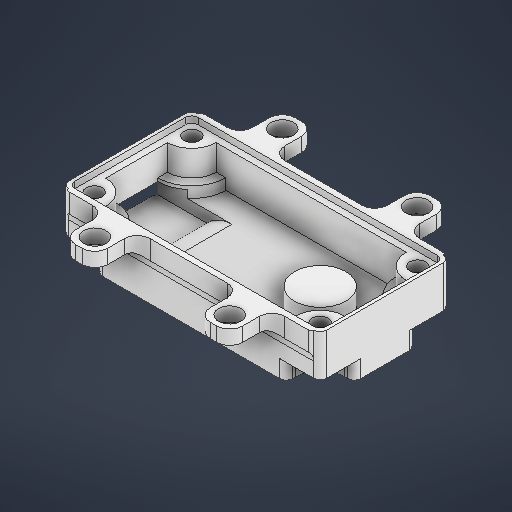
# Autodesk Inventor part: ServoCase
Saved by Autodesk Inventor 2026.2 (Build 302298010, 298A)
## iProperties
Created: 2026-02-12
Part Number: ServoCase
Material: Generic
Document SubType Name: Modeling
Designer: Liam
Density: 1 g/cm^3
Appearance: Default
Author: Liam
Autodesk Inventor part; units mm, degrees
ref_plane "YZ Plane" through (0, 0, 0) normal (1, 0, 0) x (0, 1, 0)
sketch "Sketch1" plane through (0, 0, 0) normal (0, 1, 0) x (-1, 0, 0)
  line L0 (20.1, 10.1) -> (-20.1, 10.1)
  line L1 (-20.1, 10.1) -> (-20.1, -10.1)
  line L2 (-20.1, -10.1) -> (20.1, -10.1)
  line L3 (20.1, -10.1) -> (20.1, 10.1)
  line L4 (20.1, 10.1) -> (-20.1, -10.1) construction
  line L5 (-20.1, 10.1) -> (20.1, -10.1) construction
  line L6 (-18.6, 8.6) -> (18.6, 8.6)
  line L7 (18.6, 8.6) -> (18.6, -8.6)
  line L8 (18.6, -8.6) -> (-18.6, -8.6)
  line L9 (-18.6, -8.6) -> (-18.6, 8.6)
  circle A0 centre (17.6, 7.6) radius 1.25
  line L10 (0, 0) -> (18.6, 0) construction
  line L11 (0, 0) -> (0, 0.8088) construction
  line L12 (0, 0.8088) -> (0, 8.6) construction
  circle A1 centre (17.6, -7.6) radius 1.25
  circle A2 centre (-17.6, 7.6) radius 1.25
  circle A3 centre (-17.6, -7.6) radius 1.25
  line L13 (-19.6, 9.6) -> (19.6, 9.6)
  line L14 (19.6, 9.6) -> (19.6, -9.6)
  line L15 (19.6, -9.6) -> (-19.6, -9.6)
  line L16 (-19.6, -9.6) -> (-19.6, 9.6)
  arc A4 (14.8, 8.6) -> (18.6, 4.8) centre (18.6, 8.6) ccw
  arc A5 (18.6, -4.8) -> (14.8, -8.6) centre (18.6, -8.6) ccw
  arc A6 (-18.6, 4.8) -> (-14.8, 8.6) centre (-18.6, 8.6) ccw
  arc A7 (-14.8, -8.6) -> (-18.6, -4.8) centre (-18.6, -8.6) ccw
  arc A8 (18.6, -3.3) -> (13.3, -8.6) centre (18.6, -8.6) ccw
  arc A9 (13.3, 8.6) -> (18.6, 3.3) centre (18.6, 8.6) ccw
  arc A10 (-13.3, -8.6) -> (-18.6, -3.3) centre (-18.6, -8.6) ccw
  arc A11 (-18.6, 3.3) -> (-13.3, 8.6) centre (-18.6, 8.6) ccw
  line L17 (14.8, 8.6) -> (14.8, 10.1)
  line L18 (18.6, 4.8) -> (20.1, 4.8)
  line L19 (-14.8, 8.6) -> (-14.8, 10.1)
  line L20 (-18.6, 4.8) -> (-20.1, 4.8)
  line L21 (14.8, -8.6) -> (14.8, -10.1)
  line L22 (18.6, -4.8) -> (20.1, -4.8)
  line L23 (-18.6, -4.8) -> (-20.1, -4.8)
  line L24 (-14.8, -8.6) -> (-14.8, -10.1)
  point P0 (-14.8, -8.6)
  point P1 (-18.6, -4.8)
  point P2 (-18.6, 4.8)
  point P3 (-14.8, 8.6)
  point P4 (18.6, -4.8)
  point P5 (14.8, -8.6)
  point P6 (-13.3, -8.6)
  point P7 (-18.6, -3.3)
  point P8 (-18.6, 3.3)
  point P9 (-13.3, 8.6)
  point P10 (-18.6, -4.8)
  point P11 (-18.6, 4.8)
  point P12 (-20.1, 4.8)
  point P13 (-20.1, -4.8)
  point P14 (13.3, 8.6)
  point P15 (18.6, 3.3)
  point P16 (18.6, -3.3)
  point P17 (13.3, -8.6)
  point P18 (-14.8, -8.6)
  point P19 (-14.8, -10.1)
  point P20 (14.8, -10.1)
  point P21 (20.1, -4.8)
  point P22 (-14.8, 10.1)
  point P23 (-14.8, 8.6)
  dimension "d0" = 40.2
  dimension "d1" = 20.2
  dimension "d2" = 1.5
  dimension "d3" = 2.5
  dimension "d4" = 2.5
  dimension "d5" = 2.5
  dimension "d8" = 0.5
  dimension "d9" = 3.8
  dimension "d17" = 1.5
  constraints: 50 end point, 27 symmetric about line, 16 point on circle, 12 centre point, 6 parallel, 6 perpendicular, 4 midpoint, 4 point on line, 1 coincident, 1 horizontal, 15 other
  measures "d0" distance of L1.end L2.end
  measures "d1" distance of L0.end L1.end
  measures "d2" distance between parallel lines of L6 L0
  measures "d3" diameter of A0
  measures "d4" distance from line of L3 A0.centre
  measures "d5" distance from line of L0 A0.centre
  measures "d8" distance between parallel lines of L0 L13
  measures "d9" radius of A4
  measures "d17" radial gap between concentric circles of A8 A5
extrude "Extrusion1" add sketch "Sketch1" along normal blind 6.5 contours L3 L18 L14 L13 L17 L0 | L17 L13 L19 L0 | L3 L22 L14 L18 | L19 L13 L16 L20 L1 L0 | L3 L2 L21 L15 L14 L22 | L20 L16 L23 L1 | L2 L24 L15 L21 | L23 L16 L15 L24 L2 L1
extrude "Extrusion2" add sketch "Sketch1" along normal blind 5.5 contours L17 L6 L19 L13 | L13 L14 L18 L7 A0 L6 L17 | L14 L22 L7 L18 | L19 L6 A2 L9 L20 L16 L13 | L6 A0 L7 A4 | L14 L15 L21 L8 A1 L7 L22 | A6 L9 A2 L6 | L7 A1 L8 A5 | L20 L9 L23 L16 | L6 L7 A0 | L15 L24 L8 L21 | L23 L9 A3 L8 L24 L15 L16 | A2 L9 L6 | L7 L8 A1 | A7 L8 A3 L9 | A3 L8 L9 picked at (18.5219, 8.5219) picked at (-18.5219, 8.5219) picked at (18.5219, -8.5219) picked at (-18.5219, -8.5219)
extrude "Extrusion5" add sketch "Sketch1" along normal blind 1.5 and the other way blind 2.7 contours L17 L13 L19 L0 | L3 L22 L14 L18 | L17 L6 L19 L13 | L14 L22 L7 L18 | A4 L7 A9 L6 | L20 L16 L23 L1 | L6 A11 L9 A6 | L2 L24 L15 L21 | A5 L8 A8 L7 | L20 L9 L23 L16 | L15 L24 L8 L21 | L9 A10 L8 A7
ref_plane "Work Plane1" through (0, -2.7, 0) normal (0, 1, 0) x (-1, 0, 0)
sketch "Sketch9" plane through (0, -2.7, 0) normal (0, 1, 0) x (-1, 0, 0)
  line L0 (-18.6, 4.8) -> (-20.1, 4.8) projected
  arc A0 (-14.8, -8.6) -> (-18.6, -4.8) centre (-18.6, -8.6) ccw projected
  line L1 (-20.1, 4.8) -> (-18.6, 4.8)
  line L2 (-18.6, 4.8) -> (-18.6, -4.8)
  line L3 (-18.6, -4.8) -> (-20.1, -4.8)
  line L4 (-20.1, -4.8) -> (-20.1, 4.8)
  line L5 (-14.8, -8.6) -> (-14.8, -10.1) projected
  line L6 (14.8, -10.1) -> (14.8, -8.6) projected
  line L7 (-14.8, -8.6) -> (14.8, -8.6)
  line L8 (14.8, -8.6) -> (14.8, -10.1)
  line L9 (14.8, -10.1) -> (-14.8, -10.1)
  line L10 (-14.8, -10.1) -> (-14.8, -8.6)
  line L11 (18.6, 4.8) -> (18.6, -4.8) projected
  line L12 (20.1, -10.1) -> (20.1, 10.1) projected
  line L13 (18.6, 4.8) -> (20.1, 4.8)
  line L14 (20.1, 4.8) -> (20.1, -4.8)
  line L15 (20.1, -4.8) -> (18.6, -4.8)
  line L16 (18.6, -4.8) -> (18.6, 4.8)
  line L17 (20.1, 10.1) -> (14.8, 10.1) projected
  line L18 (-14.8, 8.6) -> (-13.3, 8.6) projected
  line L19 (14.8, 10.1) -> (-14.8, 10.1)
  line L20 (-14.8, 10.1) -> (-14.8, 8.6)
  line L21 (-14.8, 8.6) -> (14.8, 8.6)
  line L22 (14.8, 8.6) -> (14.8, 10.1)
  arc A1 (-18.6, 4.8) -> (-14.8, 8.6) centre (-18.6, 8.6) ccw projected
  arc A2 (-18.6, 4.8) -> (-14.8, 8.6) centre (-18.6, 8.6) ccw
  arc A3 (-14.8, -8.6) -> (-18.6, -4.8) centre (-18.6, -8.6) ccw
  arc A4 (14.8, 8.6) -> (18.6, 4.8) centre (18.6, 8.6) ccw projected
  arc A5 (14.8, 8.6) -> (18.6, 4.8) centre (18.6, 8.6) ccw
  arc A6 (18.6, -4.8) -> (14.8, -8.6) centre (18.6, -8.6) ccw projected
  arc A7 (18.6, -4.8) -> (14.8, -8.6) centre (18.6, -8.6) ccw
  circle A8 centre (-10, 0) radius 2.5
  circle A9 centre (-10, 0) radius 4
  line L23 (-6.5, 3) -> (-3.5, 3)
  line L24 (-3.5, 3) -> (-3.5, -3)
  line L25 (-3.5, -3) -> (-6.5, -3)
  line L26 (-6.5, -3) -> (-6.5, 3)
  line L27 (-6.5, 3) -> (-3.5, -3) construction
  line L28 (-3.5, 3) -> (-6.5, -3) construction
  line L29 (-13, 3.5) -> (-13, 6.5)
  line L30 (-7, 3.5) -> (-13, 3.5)
  line L31 (-7, 6.5) -> (-7, 3.5)
  line L32 (-13, 6.5) -> (-7, 6.5)
  line L33 (-13.5, -3) -> (-16.5, -3)
  line L34 (-13.5, 3) -> (-13.5, -3)
  line L35 (-16.5, 3) -> (-13.5, 3)
  line L36 (-16.5, -3) -> (-16.5, 3)
  line L37 (-7, -3.5) -> (-7, -6.5)
  line L38 (-13, -3.5) -> (-7, -3.5)
  line L39 (-13, -6.5) -> (-13, -3.5)
  line L40 (-7, -6.5) -> (-13, -6.5)
  line L41 (12.1, -4.5) -> (15.1, -4.5)
  line L42 (15.1, -4.5) -> (15.1, 4.5)
  line L43 (15.1, 4.5) -> (12.1, 4.5)
  line L44 (12.1, 4.5) -> (12.1, -4.5)
  line L45 (12.1, -4.5) -> (15.1, 4.5) construction
  line L46 (15.1, -4.5) -> (12.1, 4.5) construction
  point P0 (0, 0)
  point P1 (18.5, 2.5)
  point P2 (20, -2.5)
  point P3 (18.5, 2.5)
  point P4 (-20.1, 0)
  point P5 (-5, 0)
  point P6 (13.6, 0)
  dimension "d58" = 5
  dimension "d59" = 10.1
  dimension "d60" = 0
  dimension "d62" = 3
  dimension "d63" = 6
  dimension "d64" = 0
  dimension "d65" = 5
  dimension "d68" = 360
  dimension "d80" = 3
  dimension "d81" = 9
  dimension "d82" = 6.5
  dimension "d83" = 10.1
  dimension "d87" = 8
  constraints: 80 end point, 12 parallel, 8 point on circle, 6 centre point, 6 horizontal, 6 perpendicular, 5 midpoint, 4 coincident, 1 point on line, 36 other
  measures "d58" diameter of A8
  measures "d59" distance from line of L4 A8.centre
  measures "d60" vertical distance of point (-20.1, 0) A8.centre
  measures "d62" distance of L24.end L25.end
  measures "d63" distance of L23.end L24.end
  measures "d64" vertical distance of point (0, 0) point (-5, 0)
  measures "d65" distance of A8.centre point (-5, 0)
  measures "d80" distance of L41.start L41.end
  measures "d81" distance of L41.end L42.end
  measures "d82" distance from line of L14 point (13.6, 0)
  measures "d83" distance from line of L19 point (13.6, 0)
  measures "d87" diameter of A9
extrude "Extrusion11" add sketch "Sketch9" along normal blind 2.5 contours A1 L18 L21 A4 L11 A6 L7 A0 L2 | A9 L26 L23 L24 L25 | A9 L30 L29 L32 L31 | L38 L37 L40 L39 A9 | A9 L34 L33 L36 L35 | L44 L43 L42 L41
extrude "Extrusion12" add sketch "Sketch9" along normal blind 5 contours A9 L26 | L26 A9 L38 L34 L30 | L30 A9 | A9 L38 | L34 A9
sketch "Sketch10" plane through (10, 2.3, 0) normal (0, 1, 0) x (1, 0, 0)
  circle A0 centre (0, 0) radius 4
  line L0 (4.8, -8.6) -> (-24.8, -8.6) projected
  line L1 (8.6, 4.8) -> (8.6, -4.8) projected
  point P0 (-10, 0)
  dimension "d72" = 8
  dimension "d74" = 8.6
  dimension "d116" = 8.6
  constraints: 1 centre point
  measures "d72" diameter of A0
  measures "d74" distance from line of L0 A0.centre
  measures "d116" distance from line of L1 A0.centre
extrude "Extrusion13" add sketch "Sketch10" along normal blind 0.5
extrude "Extrusion14" cut sketch "Sketch9" along normal blind 1.5 contours A9 L26 | A9 L26 L23 L24 L25 | L30 A9 | A9 L30 L29 L32 L31 | L38 L37 L40 L39 A9 | A9 L38 | L34 A9 | A9 L34 L33 L36 L35
fillet "Fillet5" radius 1.5 16 edges at (7, -1.95, -6.5) (7, -1.95, -3.5) (13, -1.95, -6.5) (13, -1.95, -3.5) (13.5, -1.95, -3) (16.5, -1.95, -3) (16.5, -1.95, 3) (13.5, -1.95, 3) (13, -1.95, 3.5) (13, -1.95, 6.5) (7, -1.95, 6.5) (7, -1.95, 3.5) (6.5, -1.95, 3) (3.5, -1.95, 3) (6.5, -1.95, -3) (3.5, -1.95, -3)
fillet "Fillet6" radius 1 16 edges at (20.1, 3.25, -10.1) (20.1, 3.25, 10.1) (19.6, 6, -9.6) (19.6, 6, 9.6) (-20.1, 3.25, -10.1) (-19.6, 6, -9.6) (-20.1, 3.25, 10.1) (-19.6, 6, 9.6) (-20.1, -1.35, -4.8) (-20.1, -1.35, 4.8) (-14.8, -1.35, -10.1) (-14.8, -1.35, 10.1) (14.8, -1.35, -10.1) (20.1, -1.35, -4.8) (20.1, -1.35, 4.8) (14.8, -1.35, 10.1)
sketch "Sketch11" plane through (-20.1, 0, 3.8) normal (-1, 0, 0) x (0, 0, 1)
  line L0 (-8.3, 1) -> (0.7, 1)
  line L1 (0.7, 1) -> (0.7, -2)
  line L2 (0.7, -2) -> (-8.3, -2)
  line L3 (-8.3, -2) -> (-8.3, 1)
  line L4 (-8.3, 1) -> (0.7, -2) construction
  line L5 (0.7, 1) -> (-8.3, -2) construction
  point P0 (-3.8, 0)
  point P1 (-3.8, -0.5)
  dimension "d88" = 9
  dimension "d89" = 3
  dimension "d90" = 0.5
  dimension "d91" = 0
  constraints: 12 end point, 2 midpoint, 2 parallel, 1 horizontal, 1 perpendicular
  measures "d88" distance of L1.end L2.end
  measures "d89" distance of L0.end L1.end
  measures "d90" distance of point (-3.8, 0) point (-3.8, -0.5)
  measures "d91" horizontal distance of point (-3.8, 0) point (-3.8, -0.5)
extrude "Extrusion16" cut sketch "Sketch11" against normal blind 8
ref_plane "Work Plane2" through (0, 6.5, 0) normal (0, 1, 0) x (-1, 0, 0)
sketch "Sketch12" plane through (0, 6.5, 0) normal (0, 1, 0) x (-1, 0, 0)
  circle A0 centre (-10.5, -14.6) radius 1.75
  line L0 (0, 0) -> (0, -8.6) construction
  line L1 (13.3, -8.6) -> (-13.3, -8.6) construction
  line L2 (0, 0) -> (-18.6, 0) construction
  line L3 (-19.1, -10.1) -> (19.1, -10.1) construction
  circle A1 centre (10.5, -14.6) radius 1.75
  circle A2 centre (-10.5, 14.6) radius 1.75
  circle A3 centre (10.5, 14.6) radius 1.75
  line L4 (-13, -17.1) -> (-8, -17.1)
  line L5 (-8, -17.1) -> (-8, -10.1)
  line L6 (-8, -10.1) -> (-13, -10.1)
  line L7 (-13, -10.1) -> (-13, -17.1)
  line L8 (0, -10.1) -> (-19.1, -10.1)
  line L9 (-19.1, -10.1) -> (-19.1, -10.5)
  line L10 (-19.1, -10.5) -> (0, -10.5)
  line L11 (0, -10.5) -> (0, -10.1)
  line L12 (13, -17.1) -> (8, -17.1)
  line L13 (8, -17.1) -> (8, -10.1)
  line L14 (13, -10.1) -> (13, -17.1)
  line L15 (0, -10.1) -> (19.1, -10.1)
  line L16 (19.1, -10.1) -> (19.1, -10.5)
  line L17 (19.1, -10.5) -> (0, -10.5)
  line L18 (-13, 17.1) -> (-8, 17.1)
  line L19 (-8, 17.1) -> (-8, 10.1)
  line L20 (-13, 10.1) -> (-13, 17.1)
  line L21 (0, 10.1) -> (-19.1, 10.1)
  line L22 (-19.1, 10.1) -> (-19.1, 10.5)
  line L23 (-19.1, 10.5) -> (0, 10.5)
  line L24 (8, 17.1) -> (8, 10.1)
  line L25 (13, 17.1) -> (8, 17.1)
  line L26 (13, 10.1) -> (13, 17.1)
  line L27 (19.1, 10.5) -> (0, 10.5)
  line L28 (19.1, 10.1) -> (19.1, 10.5)
  line L29 (0, 10.1) -> (19.1, 10.1)
  point P0 (-13, -10.5)
  point P1 (-8, -10.5)
  point P2 (8, -10.5)
  point P3 (13, -10.5)
  point P4 (8, 10.5)
  point P5 (-8, 10.5)
  point P6 (-13, 10.5)
  point P7 (13, 10.5)
  point P8 (13, -10.1)
  point P9 (8, -10.1)
  point P10 (-13, 10.1)
  point P11 (-8, 10.1)
  point P12 (8, 10.1)
  point P13 (13, 10.1)
  point P14 (-13, -10.1)
  dimension "d99" = 3.5
  dimension "d100" = 10.5
  dimension "d101" = 4.5
  dimension "d102" = 5
  dimension "d103" = 2.5
  dimension "d104" = 7
  dimension "d105" = 0.4
  dimension "d106" = 19.1
  dimension "d114" = 2.5
  dimension "d117" = 10.1
  dimension "d118" = 18.6
  constraints: 56 end point, 23 symmetric about line, 5 parallel, 4 centre point, 2 horizontal, 2 midpoint, 2 perpendicular, 1 point on line, 3 other
  measures "d99" diameter of A0
  measures "d100" distance from line of A0.centre L0
  measures "d101" distance from line of L3 A0.centre
  measures "d102" distance of L4.start L4.end
  measures "d103" distance from line of A0.centre L5
  measures "d104" distance between parallel lines of L3 L4
  measures "d105" distance of L8.end L9.end
  measures "d106" distance of L9.end L10.end
  measures "d114" distance from line of L4 A0.centre
  measures "d117" distance from line of L8 L2.end
  measures "d118" distance of L0.start L2.end
extrude "Extrusion18" add sketch "Sketch12" against normal blind 2.2
fillet "Fillet9" radius 2 8 edges at (-8, 5.4, 17.1) (-13, 5.4, 17.1) (8, 5.4, 17.1) (13, 5.4, 17.1) (13, 5.4, -17.1) (8, 5.4, -17.1) (-8, 5.4, -17.1) (-13, 5.4, -17.1)
fillet "Fillet11" radius 2 8 edges at (-8, 5.4, 10.5) (-13, 5.4, 10.5) (8, 5.4, 10.5) (13, 5.4, 10.5) (13, 5.4, -10.5) (8, 5.4, -10.5) (-8, 5.4, -10.5) (-13, 5.4, -10.5)
fillet "Fillet12" radius 0.5 4 edges at (-19.1, 5.4, 10.5) (19.1, 5.4, 10.5) (-19.1, 5.4, -10.5) (19.1, 5.4, -10.5)
fillet "Fillet13" radius 2 2 edges at (0, 4.3, 10.1) (0, 4.3, -10.1)
fillet "Fillet14" radius 5 1 edges at (-12.1, -0.2, 0)
equation "\"d0\" = CaseLength"
equation "\"d1\" = CaseWidth"
equation "\"d3\" = ScrewDiameter"
equation "\"d4\" = ScrewDis"
equation "\"d5\" = ScrewDis"
equation "\"CaseWidth\" = 20.2"
equation "\"CaseLength\" = 40.2"
equation "\"CaseThickness\" = 2"
equation "\"CaseScrewHeight\" = 5.5"
equation "\"CaseHeight\" = 9.2"
equation "\"ScrewDiameter\" = 2.5"
equation "\"ScrewDis\" = 2.5"
equation "\"FloorDiff\" = 2.7"
equation "\"FloorHeight\" = 2.5"
body "Solid1"
